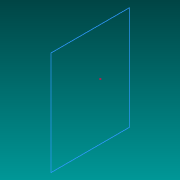
# Autodesk Inventor part: 滑块3
Saved by Autodesk Inventor 2021 (Build 250183000, 183)
## iProperties
Created: 2025-04-17
Part Number: 滑块3
Material: 常规
Document SubType Name: Modeling
Designer: 86155
Density: 1 g/cm^3
Appearance: 默认
Author: 86155
Autodesk Inventor part; units mm, degrees
ref_plane "YZ Plane" through (0, 0, 0) normal (1, 0, 0) x (0, 1, 0)
ref_plane "XZ Plane" through (0, 0, 0) normal (0, 1, 0) x (-1, 0, 0)
ref_plane "XY Plane" through (0, 0, 0) normal (0, 0, 1) x (1, 0, 0)
sketch "草图1" plane through (0, 0, 0) normal (1, 0, 0) x (0, 1, 0)
  line L0 (9.7546, -15.7991) -> (9.7546, -18.7991) projected
  line L1 (20.7546, -18.7991) -> (9.7546, -18.7991) projected
  line L2 (20.7546, -18.7991) -> (20.7546, -10.7991) projected
  line L3 (18.7546, -8.7991) -> (20.7546, -10.7991) projected
  line L4 (18.7546, -8.7991) -> (-19.2454, -8.7991) projected
  line L5 (-21.2454, -10.7991) -> (-19.2454, -8.7991) projected
  line L6 (-21.2454, -10.7991) -> (-21.2454, -18.7991) projected
  line L7 (-10.2454, -18.7991) -> (-21.2454, -18.7991) projected
  line L8 (-10.2454, -18.7991) -> (-10.2454, -15.7991) projected
  line L9 (-10.2454, -15.7991) -> (-7.2454, -15.7991) projected
  line L10 (-7.2454, -15.7991) -> (-7.2454, -13.7991) projected
  line L11 (-7.2454, -13.7991) -> (-10.2454, -13.7991) projected
  line L12 (-10.2454, -13.7991) -> (-10.2454, -10.7991) projected
  line L13 (-10.2454, -10.7991) -> (9.7546, -10.7991) projected
  line L14 (9.7546, -10.7991) -> (9.7546, -13.7991) projected
  line L15 (9.7546, -13.7991) -> (6.7546, -13.7991) projected
  line L16 (6.7546, -13.7991) -> (6.7546, -15.7991) projected
  line L17 (6.7546, -15.7991) -> (9.7546, -15.7991) projected
  line L18 (9.7546, -18.7991) -> (12.7546, -18.7991)
  line L19 (12.7546, -18.7991) -> (12.7546, -6.7991)
  line L20 (-10.2454, -18.7991) -> (-13.2454, -18.7991)
  line L21 (-13.2454, -18.7991) -> (-13.2454, -6.7991)
  line L22 (-13.2454, -6.7991) -> (12.7546, -6.7991)
  dimension "d0" = 3
  dimension "d1" = 12
  constraints: 10 end point, 2 perpendicular, 2 point on line, 1 vertical
  measures "d0" distance of L0.end L18.end
  measures "d1" distance of L18.end L19.end
extrude "拉伸1" add sketch "草图1" along normal blind 40 contours L17 L16 L15 L14 L13 L12 L11 L10 L9 L8 L7 L21 L4 L19 L1 L0 | L4 L21 L22 L19
sketch "草图2" plane through (0, -13.2454, -6.7991) normal (0, 0, 1) x (1, 0, 0)
  line L0 (40, 26) -> (40, 0) projected
  line L1 (0, 0) -> (40, 0)
  line L2 (40, 0) -> (40, 8)
  line L3 (40, 8) -> (0, 8)
  line L4 (0, 8) -> (0, 0)
  line L5 (0, 26) -> (40, 26) projected
  line L6 (0, 26) -> (40, 26)
  line L7 (40, 26) -> (40, 18)
  line L8 (40, 18) -> (0, 18)
  line L9 (0, 18) -> (0, 26)
  point P0 (0, 13.2454)
  dimension "d4" = 8
  dimension "d5" = 8
  constraints: 16 end point, 4 parallel, 2 horizontal, 2 perpendicular, 2 point on line
  measures "d4" distance of L2.end L1.end
  measures "d5" distance of L6.end L7.end
extrude "拉伸2" add sketch "草图2" along normal blind 2
